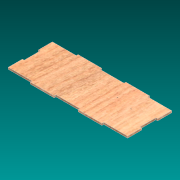
# Autodesk Inventor part: TAPA 2
Saved by Autodesk Inventor 2018 (Build 220112000, 112)
## iProperties
Created: 2019-12-06
Part Number: TAPA 2
Material: Generic
Document SubType Name: Modeling
Designer: Carlos Loaiza
Density: 1 g/cm^3
Appearance: Default
Author: Carlos Loaiza
Autodesk Inventor part; units mm, degrees
ref_plane "YZ Plane" through (0, 0, 0) normal (1, 0, 0) x (0, 1, 0)
ref_plane "XZ Plane" through (0, 0, 0) normal (0, 1, 0) x (-1, 0, 0)
ref_plane "XY Plane" through (0, 0, 0) normal (0, 0, 1) x (1, 0, 0)
sketch "Sketch1" plane through (0, 0, 0) normal (0, 0, 1) x (1, 0, 0)
  line L0 (0, 0) -> (200, 0)
  line L1 (200, 0) -> (200, 80)
  line L2 (200, 80) -> (0, 80)
  line L3 (0, 80) -> (0, 0)
  dimension "d0" = 200
  dimension "d1" = 80
  constraints: 8 end point, 3 perpendicular, 1 horizontal
  measures "d0" distance of L0.start L0.end
  measures "d1" distance of L0.end L1.end
extrude "Extrusion1" add sketch "Sketch1" along normal blind 3
sketch "Sketch2" plane through (0, 0, 3) normal (0, 0, 1) x (1, 0, 0)
  line L0 (0, 0) -> (0, 3)
  line L1 (0, 3) -> (40, 3)
  line L2 (40, 3) -> (40, 0)
  line L3 (0, 0) -> (200, 0) projected
  line L4 (40, 0) -> (80, 0)
  line L5 (80, 0) -> (80, 3)
  line L6 (80, 3) -> (120, 3)
  line L7 (120, 3) -> (120, 0)
  line L8 (120, 0) -> (160, 0)
  line L9 (160, 0) -> (160, 3)
  line L10 (160, 3) -> (200, 3)
  line L11 (0, 80) -> (0, 0) projected
  line L12 (0, 80) -> (0, 77)
  line L13 (0, 77) -> (40, 77)
  line L14 (40, 77) -> (40, 80)
  line L15 (0, 80) -> (200, 80)
  line L16 (40, 80) -> (80, 80)
  line L17 (80, 80) -> (80, 77)
  line L18 (80, 77) -> (120, 77)
  line L19 (120, 77) -> (120, 80)
  line L20 (120, 80) -> (160, 80)
  line L21 (160, 80) -> (160, 77)
  line L22 (160, 77) -> (200, 77)
  line L23 (200, 80) -> (0, 80) projected
  line L24 (0, 80) -> (0, 53.3333)
  line L25 (0, 53.3333) -> (3, 53.3333)
  line L26 (3, 53.3333) -> (3, 26.6667)
  line L27 (3, 26.6667) -> (0, 26.6667)
  line L28 (200, 53.3333) -> (197, 53.3333)
  line L29 (197, 53.3333) -> (197, 26.6667)
  line L30 (197, 26.6667) -> (200, 26.6667)
  line L31 (160, 77) -> (160, 80)
  line L32 (200, 77) -> (200, 80)
  line L33 (200, 3) -> (200, 0)
  line L34 (200, 26.6667) -> (200, 53.3333)
  dimension "d4" = 3
  dimension "d5" = 40
  dimension "d6" = 40
  dimension "d7" = 40
  dimension "d8" = 40
  dimension "d9" = 26.6667
  dimension "d10" = 3
  dimension "d11" = 26.6667
  constraints: 64 end point, 14 point on line, 7 perpendicular, 4 vertical, 2 parallel, 1 collinear
  measures "d4" distance of L0.start L0.end
  measures "d5" distance of L0.end L1.end
  measures "d6" distance of L2.end L4.end
  measures "d7" distance of L5.end L6.end
  measures "d8" distance of L7.end L8.end
  measures "d9" distance of L11.start L24.end
  measures "d10" distance of L24.end L25.end
  measures "d11" distance of L25.end L26.end
extrude "Extrusion2" cut sketch "Sketch2" against normal blind 3
body "Solid1"
